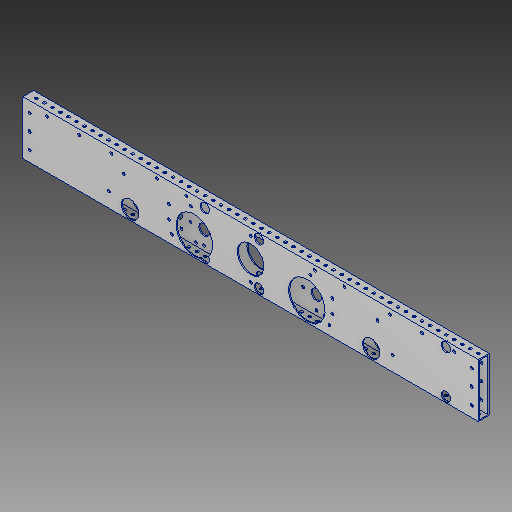
# Autodesk Inventor part: Side Extrusion
Saved by Autodesk Inventor 2019.4 (Build 234330000, 330)
## iProperties
Created: 2019-11-02
Part Number: Side Extrusion
Material: Aluminum 6061
Document SubType Name: Modeling
Designer: admin
Density: 2.7 g/cm^3
Appearance: Aluminum - Flat
Mass: 944.762 g
Surface Area: 3612.85 cm^2
Volume: 349.912 cm^3
Author: admin
Autodesk Inventor part; units mm, degrees
ref_plane "YZ Plane" through (0, 0, 0) normal (1, 0, 0) x (0, 1, 0)
ref_plane "XZ Plane" through (0, 0, 0) normal (0, 1, 0) x (-1, 0, 0)
ref_plane "XY Plane" through (0, 0, 0) normal (0, 0, 1) x (1, 0, 0)
sketch "Sketch1" plane through (0, 0, 0) normal (1, 0, 0) x (0, 1, 0)
  line L0 (-50, 10) -> (50, 10)
  line L1 (50, 10) -> (50, -10)
  line L2 (50, -10) -> (-50, -10)
  line L3 (-50, -10) -> (-50, 10)
  line L4 (-50, 10) -> (50, -10) construction
  line L5 (50, 10) -> (-50, -10) construction
  line L6 (48, -8) -> (48, 8)
  line L7 (48, 8) -> (-48, 8)
  line L8 (-48, 8) -> (-48, -8)
  line L9 (-48, -8) -> (48, -8)
  point P0 (0, 0)
  dimension "d0" = 100
  dimension "d1" = 20
  dimension "d2" = 2
  constraints: 20 end point, 4 parallel, 2 midpoint, 2 perpendicular, 1 horizontal, 3 other
  measures "d0" distance of L1.end L2.end
  measures "d1" distance of L0.end L1.end
  measures "d2" distance between parallel lines of L1 L6
extrude "Extrusion1" add sketch "Sketch1" along normal blind 850
sketch "Sketch2" plane through (0, -50, 10) normal (0, 0, -1) x (-1, 0, 0)
  circle A0 centre (-200, 18.3) radius 16.3
  line L0 (0, 0) -> (-850, 0) projected
  line L1 (0, 100) -> (0, 0) projected
  line L2 (0, 100) -> (-850, 100) projected
  line L3 (0, 0) -> (-850, 0) projected
  circle A1 centre (-650, 18.3) radius 16.3
  line L4 (-850, 100) -> (-850, 0) projected
  point P0 (0, 50)
  dimension "d5" = 32.6
  dimension "d9" = 200
  dimension "d113" = 200
  constraints: 2 centre point
  measures "d5" diameter of A0
  measures "d9" distance from line of L1 A0.centre
  measures "d113" distance from line of L4 A1.centre
extrude "Extrusion2" cut sketch "Sketch2" along normal blind 2 contours A0 | A1
sketch "Sketch3" plane through (0, -50, 10) normal (0, 0, 1) x (1, 0, 0)
  circle A0 centre (320, 36) radius 34
  line L0 (0, 0) -> (0, 100) projected
  line L1 (0, 0) -> (850, 0) projected
  line L2 (425, 100) -> (425, 0)
  circle A1 centre (530, 36) radius 34
  point P0 (0, 50)
  dimension "d10" = 68
  dimension "d11" = 320
  dimension "d12" = 36
  constraints: 2 centre point, 2 end point, 1 midpoint, 1 symmetric about line, 1 other
  measures "d10" diameter of A0
  measures "d11" distance from line of L0 A0.centre
  measures "d12" distance from line of A0.centre L1
extrude "Extrusion3" cut sketch "Sketch3" against normal blind 2
sketch "Sketch4" plane through (0, -50, -10) normal (0, 0, -1) x (-1, 0, 0)
  circle A0 centre (-200, 18.3) radius 16.3 construction
  circle A1 centre (-200, 18.3) radius 16.3 construction
  circle A2 centre (-200, 18.3) radius 12.3
  line L0 (0, 0) -> (-850, 0) projected
  line L1 (-425, 0) -> (-425, 100)
  line L2 (0, 100) -> (-850, 100) projected
  circle A3 centre (-650, 18.3) radius 12.3
  point P0 (0, 50)
  point P1 (-200, 2)
  dimension "d17" = 24.6
  constraints: 2 centre point, 2 end point, 2 midpoint, 1 coincident, 1 symmetric about line, 1 vertical alignment, 1 other
  measures "d17" diameter of A2
extrude "Extrusion4" cut sketch "Sketch4" against normal blind 2
sketch "Sketch5" plane through (0, -50, -10) normal (0, 0, -1) x (-1, 0, 0)
  circle A0 centre (-216, 18.3) radius 2.25
  circle A1 centre (-200, 18.3) radius 12.3 projected
  line L0 (-200, 18.3) -> (-216, 18.3) construction
  circle A2 centre (-200, 34.3) radius 2.25
  circle A3 centre (-184, 18.3) radius 2.25
  line L1 (0, 100) -> (-850, 100) projected
  line L2 (-425, 100) -> (-425, 0)
  line L3 (0, 0) -> (-850, 0) projected
  circle A4 centre (-634, 18.3) radius 2.25
  circle A5 centre (-650, 34.3) radius 2.25
  circle A6 centre (-666, 18.3) radius 2.25
  point P0 (0, 50)
  dimension "d18" = 4.5
  dimension "d21" = 16
  dimension "d24" = 180
  constraints: 6 centre point, 4 end point, 3 symmetric about line, 2 midpoint, 1 horizontal, 8 other
  measures "d18" diameter of A0
  measures "d21" distance of L0.start L0.end
extrude "Extrusion5" cut sketch "Sketch5" against normal blind 2 contours A0 | A2 | A3 | A4 | A5 | A6
sketch "Sketch6" plane through (0, -50, -10) normal (0, 0, -1) x (-1, 0, 0)
  circle A0 centre (-320, 36) radius 10
  line L0 (0, 0) -> (-850, 0)
  line L1 (0, 100) -> (0, 0)
  circle A1 centre (-320, 36) radius 25.4
  circle A2 centre (-320, 61.4) radius 2.75
  circle A3 centre (-345.4, 36) radius 2.75
  circle A4 centre (-320, 10.6) radius 2.75
  circle A5 centre (-294.6, 36) radius 2.75
  line L2 (-253.104106, 23.400764) -> (-232.795044, 42.581828)
  arc A6 (-232.795044, 42.581828) -> (-221.861202, 43.200848) centre (-228.087042, 56.296226) ccw
  line L3 (-221.861202, 43.200848) -> (-214.225519, 31.637858)
  arc A7 (-214.225519, 31.637858) -> (-219.215212, 21.622298) centre (-200.000275, 18.300226) ccw
  line L4 (-219.215212, 21.622298) -> (-250.723733, 18.236908)
  arc A8 (-253.104106, 23.400764) -> (-250.723733, 18.236908) centre (-251.04422, 21.21974) ccw
  line L5 (-211.588609, 53.460841) -> (-194.873767, 53.460841)
  arc A9 (-192.370348, 52.113987) -> (-194.873767, 53.460841) centre (-194.873767, 50.460841) ccw
  line L6 (-192.370348, 52.113987) -> (-179.138449, 32.076445)
  arc A10 (-175.035626, 16.971193) -> (-179.138449, 32.076445) centre (-200.000275, 18.300226) ccw
  arc A11 (-178.031384, 14.130677) -> (-175.035626, 16.971193) centre (-178.031384, 17.130677) ccw
  arc A12 (-180.528551, 17.250469) -> (-178.031384, 14.130677) centre (-177.532902, 17.088968) ccw
  arc A13 (-180.528551, 17.250469) -> (-207.029984, 36.489046) centre (-200.000275, 18.300226) ccw
  arc A14 (-210.536046, 37.520558) -> (-207.029984, 36.489046) centre (-208.111478, 39.287326) ccw
  line L7 (-210.536046, 37.520558) -> (-215.905928, 44.889746)
  arc A15 (-215.985191, 48.309036) -> (-215.905928, 44.889746) centre (-213.481359, 46.656514) ccw
  arc A16 (-215.985191, 48.309036) -> (-214.416912, 51.461193) centre (-228.087042, 56.296226) ccw
  arc A17 (-211.588609, 53.460841) -> (-214.416912, 51.461193) centre (-211.588609, 50.460841) ccw
  line L8 (-284.480973, 40.652695) -> (-284.222617, 32.873773)
  arc A18 (-288.433061, 30.029957) -> (-284.222617, 32.873773) centre (-287.220964, 32.774191) ccw
  line L9 (-288.433061, 30.029957) -> (-290.947932, 31.140747)
  arc A19 (-305.816396, 47.278292) -> (-290.947932, 31.140747) centre (-279.837042, 56.296226) ccw
  arc A20 (-302.982285, 51.262067) -> (-305.816396, 47.278292) centre (-302.982285, 48.262067) ccw
  line L10 (-302.982285, 51.262067) -> (-295.383819, 51.262067)
  arc A21 (-292.718657, 49.639351) -> (-295.383819, 51.262067) centre (-295.383819, 48.262067) ccw
  arc A22 (-292.718657, 49.639351) -> (-286.169215, 43.251933) centre (-279.837042, 56.296226) ccw
  arc A23 (-284.480973, 40.652695) -> (-286.169215, 43.251933) centre (-287.479319, 40.553113) ccw
  arc A24 (-214.415926, -2.662574) -> (-211.443355, 2.510802) centre (-213.203829, 0.08166) ccw
  line L11 (-214.415926, -2.662574) -> (-233.317299, 5.685948)
  arc A25 (-232.531596, 11.399725) -> (-233.317299, 5.685948) centre (-232.105201, 8.430182) ccw
  line L12 (-232.531596, 11.399725) -> (-221.353674, 13.004754)
  arc A26 (-218.137012, 11.137213) -> (-221.353674, 13.004754) centre (-220.927279, 10.035211) ccw
  arc A27 (-218.137012, 11.137213) -> (-211.443355, 2.510802) centre (-200.000275, 18.300226) ccw
  arc A28 (-192.284251, 0.391765) -> (-193.492561, -1.479829) centre (-191.492864, -1.445001) ccw
  arc A29 (-192.284251, 0.391765) -> (-186.463613, 4.264244) centre (-200.000275, 18.300226) ccw
  arc A30 (-185.075238, 4.824656) -> (-186.463613, 4.264244) centre (-185.075238, 2.824656) ccw
  arc A31 (-181.505821, 1.478954) -> (-182.985377, 4.824656) centre (-182.985377, 2.824656) ccw
  arc A32 (-190.722566, -4.914513) -> (-181.505821, 1.478954) centre (-200.000275, 18.300226) ccw
  line L13 (-284.545044, 79.552122) -> (-284.545044, 72.007264)
  arc A33 (-286.223672, 69.313943) -> (-284.545044, 72.007264) centre (-287.545044, 72.007264) ccw
  arc A34 (-286.223672, 69.313943) -> (-292.718657, 62.9531) centre (-279.837042, 56.296226) ccw
  arc A35 (-295.383819, 61.330385) -> (-292.718657, 62.9531) centre (-295.383819, 64.330385) ccw
  line L14 (-295.383819, 61.330385) -> (-302.982285, 61.330385)
  arc A36 (-305.816396, 65.314159) -> (-302.982285, 61.330385) centre (-302.982285, 64.330385) ccw
  arc A37 (-288.48888, 82.399783) -> (-305.816396, 65.314159) centre (-279.837042, 56.296226) ccw
  arc A38 (-284.545044, 79.552122) -> (-288.48888, 82.399783) centre (-287.545044, 79.552122) ccw
  line L15 (-228.585112, 83.796226) -> (-228.087042, 83.796226)
  arc A39 (-205.139033, 71.450067) -> (-228.087042, 83.796226) centre (-228.087042, 56.296226) ccw
  line L16 (-205.139033, 71.450067) -> (-200.077204, 63.784757)
  arc A40 (-202.580623, 59.131611) -> (-200.077204, 63.784757) centre (-202.580623, 62.131611) ccw
  line L17 (-202.580623, 59.131611) -> (-211.588609, 59.131611)
  arc A41 (-214.416912, 61.131259) -> (-211.588609, 59.131611) centre (-211.588609, 62.131611) ccw
  arc A42 (-214.416912, 61.131259) -> (-226.31563, 70.687616) centre (-228.087042, 56.296226) ccw
  arc A43 (-228.763039, 72.624992) -> (-226.31563, 70.687616) centre (-225.949131, 73.665144) ccw
  line L18 (-228.763039, 72.624992) -> (-231.399021, 79.756073)
  arc A44 (-228.585112, 83.796226) -> (-231.399021, 79.756073) centre (-228.585112, 80.796226) ccw
  line L19 (-265.847311, 52.483428) -> (-242.076773, 52.483428)
  arc A45 (-242.076773, 52.483428) -> (-238.294776, 45.998062) centre (-228.087042, 56.296226) ccw
  line L20 (-238.294776, 45.998062) -> (-267.247335, 24.919745)
  arc A46 (-271.929703, 26.642844) -> (-267.247335, 24.919745) centre (-269.013051, 27.34508) ccw
  line L21 (-271.929703, 26.642844) -> (-275.109946, 39.851591)
  arc A47 (-273.50365, 43.252524) -> (-275.109946, 39.851591) centre (-272.193293, 40.553828) ccw
  arc A48 (-273.50365, 43.252524) -> (-265.847311, 52.483428) centre (-279.837042, 56.296226) ccw
  line L22 (-244.206464, 60.109024) -> (-263.717619, 60.109024)
  arc A49 (-266.480949, 61.941115) -> (-263.717619, 60.109024) centre (-263.717619, 63.109024) ccw
  arc A50 (-266.480949, 61.941115) -> (-271.460037, 68.131588) centre (-279.837042, 56.296226) ccw
  arc A51 (-272.726863, 70.580283) -> (-271.460037, 68.131588) centre (-269.726863, 70.580283) ccw
  line L23 (-272.726863, 70.580283) -> (-272.726863, 80.796226)
  arc A52 (-269.726863, 83.796226) -> (-272.726863, 80.796226) centre (-269.726863, 80.796226) ccw
  line L24 (-269.726863, 83.796226) -> (-241.992001, 83.796226)
  arc A53 (-239.348967, 82.215513) -> (-241.992001, 83.796226) centre (-241.992001, 80.796226) ccw
  line L25 (-239.348967, 82.215513) -> (-234.298397, 72.810208)
  arc A54 (-235.423535, 68.803259) -> (-234.298397, 72.810208) centre (-236.94143, 71.390921) ccw
  arc A55 (-235.423535, 68.803259) -> (-241.443135, 61.941115) centre (-228.087042, 56.296226) ccw
  arc A56 (-244.206464, 60.109024) -> (-241.443135, 61.941115) centre (-244.206464, 63.109024) ccw
  circle A57 centre (-188.087042, 69.219) radius 2.75
  circle A58 centre (-277.837042, 16.582759) radius 2.75
  circle A59 centre (-250.087042, 92.776017) radius 2.75
  circle A60 centre (-160.000305, 27.300362) radius 2.75
  circle A61 centre (-313.422276, 79.81286) radius 2.75
  circle A62 centre (-200.000275, 18.300226) radius 9.5
  circle A63 centre (-228.087042, 56.296226) radius 9.5
  circle A64 centre (-279.837042, 56.296226) radius 9.5
  arc A65 (-244.094047, 93.065872) -> (-256.080036, 92.486162) centre (-250.087042, 92.776017) ccw
  line L26 (-256.080036, 92.486162) -> (-281.527863, 91.255361)
  arc A66 (-281.527863, 91.255361) -> (-302.063851, 83.332663) centre (-279.837042, 56.296226) ccw
  line L27 (-312.063851, 85.657061) -> (-302.063851, 83.332663)
  arc A67 (-312.063851, 85.657061) -> (-318.449419, 76.537524) centre (-313.422276, 79.81286) ccw
  line L28 (-312.844999, 67.935588) -> (-318.449419, 76.537524)
  arc A68 (-312.844999, 67.935588) -> (-294.877776, 24.692804) centre (-279.837042, 56.296226) ccw
  line L29 (-294.877776, 24.692804) -> (-283.254771, 19.16117)
  arc A69 (-283.254771, 19.16117) -> (-272.419312, 14.004347) centre (-277.837042, 16.582759) ccw
  line L30 (-272.419312, 14.004347) -> (-215.041009, -13.303196)
  arc A70 (-215.041009, -13.303196) -> (-165.000275, 18.300352) centre (-200.000275, 18.300226) ccw
  line L31 (-160.000305, 21.300362) -> (-162.000275, 21.300362)
  arc A71 (-160.000305, 21.300362) -> (-156.580779, 22.370166) centre (-160.000305, 27.300362) ccw
  arc A72 (-169.897664, 36.156116) -> (-170.793719, 37.586933) centre (-200.000275, 18.300226) ccw
  line L32 (-170.793719, 37.586933) -> (-184.354376, 58.122326)
  arc A73 (-187.633238, 75.201814) -> (-191.393334, 74.225838) centre (-188.087042, 69.219) ccw
  line L33 (-195.5499, 75.076111) -> (-196.794303, 76.960555)
  arc A74 (-196.794303, 76.960555) -> (-229.898636, 93.752442) centre (-228.087042, 56.296226) ccw
  line L34 (-229.898636, 93.752442) -> (-244.094047, 93.065872)
  line L35 (0, 100) -> (-850, 100)
  line L36 (-425, 100) -> (-425, 0)
  circle A75 centre (-530, 61.4) radius 2.75
  circle A76 centre (-504.6, 36) radius 2.75
  circle A77 centre (-530, 10.6) radius 2.75
  circle A78 centre (-555.4, 36) radius 2.75
  circle A79 centre (-661.912958, 69.219) radius 2.75
  circle A80 centre (-572.162958, 16.582759) radius 2.75
  circle A81 centre (-599.912958, 92.776017) radius 2.75
  circle A82 centre (-689.999695, 27.300362) radius 2.75
  circle A83 centre (-536.577724, 79.81286) radius 2.75
  line L37 (-156.580779, 22.370166) -> (-137.281762, 35.755737)
  arc A84 (-137.281762, 35.755737) -> (-147.167505, 72.132439) centre (-148.680183, 52.189726) ccw
  line L38 (-147.167505, 72.132439) -> (-187.633238, 75.201814)
  arc A85 (-195.5499, 75.076111) -> (-191.393334, 74.225838) centre (-193.046481, 76.729257) ccw
  arc A86 (-162.000275, 21.300362) -> (-165.000275, 18.300352) centre (-162.000275, 18.300362) ccw
  circle A87 centre (-148.680183, 52.189726) radius 10.5
  circle A88 centre (-163.234444, 48.560195) radius 1.65
  arc A89 (-181.624055, 62.766879) -> (-184.354376, 58.122326) centre (-181.850957, 59.775472) ccw
  line L39 (-181.624055, 62.766879) -> (-170.444252, 61.918877)
  arc A90 (-167.802767, 58.048634) -> (-170.444252, 61.918877) centre (-170.671154, 58.92747) ccw
  arc A91 (-167.802767, 58.048634) -> (-164.446092, 39.883788) centre (-148.680183, 52.189726) ccw
  arc A92 (-165.101215, 35.572799) -> (-164.446092, 39.883788) centre (-166.810978, 38.037897) ccw
  line L40 (-165.101215, 35.572799) -> (-165.607677, 35.221523)
  arc A93 (-169.897664, 36.156116) -> (-165.607677, 35.221523) centre (-167.31744, 37.686621) ccw
  circle A94 centre (-144.546319, 66.608851) radius 1.65
  circle A95 centre (-138.259787, 41.400132) radius 1.65
  circle A96 centre (-530, 36) radius 10
  line L41 (-193.464479, -3.092162) -> (-193.492561, -1.479829)
  line L42 (-185.075238, 4.824656) -> (-182.985377, 4.824656)
  arc A97 (-193.464479, -3.092162) -> (-190.722566, -4.914513) centre (-191.464783, -3.057334) ccw
  point P0 (0, 50)
  point P1 (-200.000275, 18.300226)
  point P2 (-200.000275, 18.300226)
  point P3 (-200.000275, 18.300226)
  point P4 (-200.000275, 18.300226)
  point P5 (-162.000275, 18.300362)
  point P6 (-167.31744, 37.686621)
  point P7 (-200.000275, 18.300226)
  dimension "d31" = 50.8
  dimension "d28" = 20
  dimension "d29" = 36
  dimension "d30" = 320
  dimension "d32" = 5.5
  dimension "d35" = 360
  dimension "d46" = 36
  constraints: 15 centre point, 10 symmetric about line, 2 end point, 2 midpoint, 1 coincident, 1 vertical alignment, 21 other
  measures "d28" diameter of A0
  measures "d29" distance from line of L0 A0.centre
  measures "d30" distance from line of L1 A0.centre
  measures "d32" diameter of A2
  measures "d46" distance from line of L0 A3.centre
extrude "Extrusion6" cut sketch "Sketch6" against normal blind 50 contours A0 | A2 A1 | A1 A2 | A4 A1 | A1 A4 | A5 A1 | A1 A5 A19 | A5 A19 | A3 A1 | A1 A3 | A57 | A58 | A59 | A60 | A61 | A75 | A76 | A77 | A78 | A79 | A80 | A81 | A82 | A83 | A96 picked at (-296.100043, 35.292408)
sketch "Sketch7" plane through (0, -50, -10) normal (0, 0, -1) x (-1, 0, 0)
  circle A0 centre (-228.087, 56.296) radius 10.5
  line L0 (0, 100) -> (-850, 100) projected
  line L1 (0, 100) -> (0, 0) projected
  circle A1 centre (-279.787, 56.296) radius 10.5
  line L2 (-228.087, 56.296) -> (-279.787, 56.296) construction
  line L3 (-425, 100) -> (-425, 0)
  circle A2 centre (-621.913, 56.296) radius 10.5
  circle A3 centre (-570.213, 56.296) radius 10.5
  point P0 (0, 50)
  dimension "d39" = 43.704
  dimension "d40" = 228.087
  dimension "d41" = 21
  dimension "d44" = 21
  dimension "d45" = 51.7
  constraints: 4 centre point, 4 end point, 2 symmetric about line, 1 horizontal, 1 midpoint, 1 vertical, 2 other
  measures "d39" distance from line of L0 L2.start
  measures "d40" distance from line of L1 L2.start
  measures "d41" diameter of A0
  measures "d44" diameter of A1
  measures "d45" distance of L2.start L2.end
extrude "Extrusion7" cut sketch "Sketch7" against normal up to surface (2 mm away)
sketch "Sketch8" plane through (0, -50, -10) normal (0, 0, -1) x (-1, 0, 0)
  circle A0 centre (-425, 87.5) radius 2.75
  circle A1 centre (-545, 92) radius 2.75
  circle A2 centre (-685, 90.5) radius 2.75
  circle A3 centre (-805, 90.5) radius 2.75
  circle A4 centre (-745, 90.5) radius 2.75
  circle A5 centre (-837.5, 50) radius 2.75
  circle A6 centre (-837.5, 80) radius 2.75
  circle A7 centre (-837.5, 20) radius 2.75
  circle A8 centre (-425, 12.5) radius 2.75
  circle A9 centre (-545, 8) radius 2.75
  line L0 (-850, 0) -> (-850, 100) construction
  line L1 (0, 100) -> (-850, 100) construction
  line L2 (0, 0) -> (-850, 0) construction
  line L3 (0, 0) -> (-850, 0) construction
  line L4 (-425, 0) -> (-425, 100)
  circle A10 centre (-305, 92) radius 2.75
  circle A11 centre (-165, 90.5) radius 2.75
  circle A12 centre (-45, 90.5) radius 2.75
  circle A13 centre (-105, 90.5) radius 2.75
  circle A14 centre (-12.5, 50) radius 2.75
  circle A15 centre (-12.5, 80) radius 2.75
  circle A16 centre (-12.5, 20) radius 2.75
  circle A17 centre (-305, 8) radius 2.75
  line L5 (0, 0) -> (0, 100) construction
  line L6 (0, 0) -> (-850, 0) construction
  line L7 (0, 0) -> (-850, 0) projected
  line L8 (0, 100) -> (0, 0) projected
  line L9 (-850, 0) -> (-850, 100) projected
  dimension "d49" = 5.5
  dimension "d50" = 5.5
  dimension "d51" = 5.5
  dimension "d52" = 12.5
  dimension "d53" = 12.5
  dimension "d54" = 12.5
  dimension "d55" = 20
  dimension "d56" = 20
  dimension "d57" = 50
  dimension "d58" = 45
  dimension "d59" = 105
  dimension "d60" = 60
  dimension "d61" = 9.5
  dimension "d62" = 9.5
  dimension "d63" = 9.5
  dimension "d64" = 5.5
  dimension "d65" = 5.5
  dimension "d66" = 5.5
  dimension "d80" = 12.5
  dimension "d81" = 8
  dimension "d84" = 8
  dimension "d88" = 305
  dimension "d89" = 305
  dimension "d90" = 12.5
  dimension "d91" = 100
  dimension "d133" = 90
  constraints: 18 centre point, 14 end point, 8 symmetric about line, 4 equal radius, 3 collinear, 3 point on line, 2 midpoint, 8 other
  measures "d49" diameter of A6
  measures "d50" diameter of A5
  measures "d51" diameter of A7
  measures "d52" distance from line of L0 A7.centre
  measures "d53" distance from line of L0 A5.centre
  measures "d54" distance from line of L0 A6.centre
  measures "d55" distance from line of L1 A6.centre
  measures "d56" distance from line of L2 A7.centre
  measures "d57" distance from line of L1 A5.centre
  measures "d58" distance from line of L0 A3.centre
  measures "d59" distance from line of L0 A4.centre
  measures "d60" distance of A4.centre A2.centre
  measures "d61" distance from line of L1 A3.centre
  measures "d62" distance from line of L1 A4.centre
  measures "d63" distance from line of L1 A2.centre
  measures "d64" diameter of A3
  measures "d65" diameter of A4
  measures "d66" diameter of A2
  measures "d80" distance from line of L2 A8.centre
  measures "d81" distance from line of L2 A9.centre
  measures "d84" distance from line of L1 A1.centre
  measures "d88" distance from line of L0 A1.centre
  measures "d89" distance from line of L0 A9.centre
  measures "d90" distance from line of L1 A0.centre
  measures "d91" distance between parallel lines of L1 L3
  measures "d133" angle of L1 L5
extrude "Extrusion8" cut sketch "Sketch8" against normal blind 50
sketch "Sketch9" plane through (0, -50, 10) normal (0, 0, 1) x (1, 0, 0)
  circle A0 centre (272.5, 62.5) radius 2.75
  circle A1 centre (272.5, 37.5) radius 2.75
  line L0 (0, 100) -> (850, 100) projected
  line L1 (425, 100) -> (425, 0)
  line L2 (0, 0) -> (850, 0) projected
  line L3 (0, 0) -> (0, 100) projected
  circle A2 centre (577.5, 62.5) radius 2.75
  circle A3 centre (577.5, 37.5) radius 2.75
  point P0 (0, 50)
  dimension "d94" = 5.5
  dimension "d95" = 5.5
  dimension "d96" = 272.5
  dimension "d97" = 272.5
  dimension "d98" = 37.5
  dimension "d99" = 37.5
  constraints: 4 centre point, 2 end point, 2 midpoint, 2 symmetric about line, 2 other
  measures "d94" diameter of A0
  measures "d95" diameter of A1
  measures "d96" distance from line of L3 A0.centre
  measures "d97" distance from line of L3 A1.centre
  measures "d98" distance from line of L2 A1.centre
  measures "d99" distance from line of L0 A0.centre
extrude "Extrusion9" cut sketch "Sketch9" against normal blind 5 contours A0 | A1 | A2 | A3
sketch "Sketch10" plane through (0, 50, 10) normal (0, 1, 0) x (1, 0, 0)
  line L0 (0, 20) -> (850, 20) projected
  circle A0 centre (15, 10) radius 2.75
  line L1 (15, 10) -> (0, 10) construction
  circle A1 centre (30, 10) radius 2.75
  circle A2 centre (45, 10) radius 2.75
  circle A3 centre (60, 10) radius 2.75
  circle A4 centre (75, 10) radius 2.75
  circle A5 centre (90, 10) radius 2.75
  circle A6 centre (105, 10) radius 2.75
  circle A7 centre (120, 10) radius 2.75
  circle A8 centre (135, 10) radius 2.75
  circle A9 centre (150, 10) radius 2.75
  circle A10 centre (165, 10) radius 2.75
  circle A11 centre (180, 10) radius 2.75
  circle A12 centre (195, 10) radius 2.75
  circle A13 centre (210, 10) radius 2.75
  circle A14 centre (225, 10) radius 2.75
  circle A15 centre (240, 10) radius 2.75
  circle A16 centre (255, 10) radius 2.75
  circle A17 centre (270, 10) radius 2.75
  circle A18 centre (285, 10) radius 2.75
  circle A19 centre (300, 10) radius 2.75
  circle A20 centre (315, 10) radius 2.75
  circle A21 centre (330, 10) radius 2.75
  circle A22 centre (345, 10) radius 2.75
  circle A23 centre (360, 10) radius 2.75
  circle A24 centre (375, 10) radius 2.75
  circle A25 centre (390, 10) radius 2.75
  circle A26 centre (405, 10) radius 2.75
  circle A27 centre (420, 10) radius 2.75
  circle A28 centre (435, 10) radius 2.75
  circle A29 centre (450, 10) radius 2.75
  circle A30 centre (465, 10) radius 2.75
  circle A31 centre (480, 10) radius 2.75
  circle A32 centre (495, 10) radius 2.75
  circle A33 centre (510, 10) radius 2.75
  circle A34 centre (525, 10) radius 2.75
  circle A35 centre (540, 10) radius 2.75
  circle A36 centre (555, 10) radius 2.75
  circle A37 centre (570, 10) radius 2.75
  circle A38 centre (585, 10) radius 2.75
  circle A39 centre (600, 10) radius 2.75
  circle A40 centre (615, 10) radius 2.75
  circle A41 centre (630, 10) radius 2.75
  circle A42 centre (645, 10) radius 2.75
  circle A43 centre (660, 10) radius 2.75
  circle A44 centre (675, 10) radius 2.75
  circle A45 centre (690, 10) radius 2.75
  circle A46 centre (705, 10) radius 2.75
  circle A47 centre (720, 10) radius 2.75
  circle A48 centre (735, 10) radius 2.75
  circle A49 centre (750, 10) radius 2.75
  circle A50 centre (765, 10) radius 2.75
  circle A51 centre (780, 10) radius 2.75
  circle A52 centre (795, 10) radius 2.75
  circle A53 centre (810, 10) radius 2.75
  circle A54 centre (825, 10) radius 2.75
  circle A55 centre (840, 10) radius 2.75
  dimension "d102" = 5.5
  dimension "d103" = 15
  dimension "d106" = 15
  constraints: 56 centre point, 2 end point, 2 horizontal, 110 other
  measures "d102" diameter of A0
  measures "d103" distance of L1.start L1.end
  measures "d106" distance of L1.start A1.centre
extrude "Extrusion10" cut sketch "Sketch10" against normal through all
sketch "Sketch11" plane through (0, -50, -10) normal (0, 0, -1) x (-1, 0, 0)
  point P0 (0, 50)
sketch "Sketch12" plane through (0, -50, -10) normal (0, 0, -1) x (-1, 0, 0)
  circle A0 centre (-577.5, 62.5) radius 2.75 projected
  circle A1 centre (-577.5, 62.5) radius 2.75 projected
  circle A2 centre (-577.5, 37.5) radius 2.75 projected
  circle A3 centre (-577.5, 37.5) radius 2.75 projected
  circle A4 centre (-272.5, 62.5) radius 2.75 projected
  circle A5 centre (-272.5, 62.5) radius 2.75 projected
  circle A6 centre (-272.5, 37.5) radius 2.75 projected
  circle A7 centre (-272.5, 37.5) radius 2.75 projected
  circle A8 centre (-577.5, 37.5) radius 7.5
  circle A9 centre (-272.5, 37.5) radius 7.5
  point P0 (0, 50)
  dimension "d114" = 15
  dimension "d115" = 15
  constraints: 2 centre point, 2 coincident
  measures "d114" diameter of A8
  measures "d115" diameter of A9
extrude "Extrusion11" cut sketch "Sketch12" against normal blind 2 contours A2 | A6 | A8 | A9
sketch "Sketch13" plane through (0, -50, -10) normal (0, 0, -1) x (-1, 0, 0)
  circle A0 centre (-789.4, 90) radius 2.75 projected
  circle A1 centre (-789.5, 10) radius 2.75 projected
  circle A2 centre (-440.6, 90) radius 2.75 projected
  circle A3 centre (-440.6, 10) radius 2.75 projected
  circle A4 centre (-339.4, 90) radius 2.75 projected
  circle A5 centre (-339.4, 10) radius 2.75 projected
  point P0 (0, 50)
extrude "Extrusion12" cut sketch "Sketch13" against normal through all
sketch "Sketch14" plane through (0, -50, 10) normal (0, 0, 1) x (1, 0, 0)
  circle A0 centre (339.4, 90) radius 2.75
  circle A1 centre (789.4, 90) radius 2.75
  circle A2 centre (789.5, 10) radius 2.75
  circle A3 centre (440.6, 10) radius 2.75
  circle A4 centre (440.6, 90) radius 2.75
  circle A5 centre (339.4, 90) radius 2.75
  circle A6 centre (339.4, 10) radius 2.75
  circle A7 centre (339.4, 90) radius 8.75
  circle A8 centre (339.4, 10) radius 8.75
  circle A9 centre (440.6, 10) radius 8.75
  circle A10 centre (440.6, 90) radius 8.75
  circle A11 centre (789.4, 90) radius 8.75
  circle A12 centre (789.5, 10) radius 8.75
  point P0 (0, 50)
extrude "Extrusion13" cut sketch "Sketch14" against normal blind 3
sketch "Sketch15" plane through (0, -50, -10) normal (0, 0, -1) x (-1, 0, 0)
  circle A0 centre (-425, 50) radius 25
  line L0 (0, 0) -> (-850, 0) projected
  line L1 (0, 100) -> (0, 0) projected
  point P0 (0, 50)
  dimension "d128" = 50
  dimension "d129" = 50
  dimension "d130" = 425
  constraints: 1 centre point
  measures "d128" diameter of A0
  measures "d129" distance from line of L0 A0.centre
  measures "d130" distance from line of L1 A0.centre
extrude "Extrusion14" cut sketch "Sketch15" against normal blind 65.5
sketch "Sketch16" plane through (0, -50, -10) normal (0, 0, -1) x (-1, 0, 0)
  circle A0 centre (-425, 12.5) radius 2.75 projected
  circle A1 centre (-425, 12.5) radius 7.75
  point P0 (0, 50)
  dimension "d134" = 5
  constraints: 1 centre point
  measures "d134" radial gap between concentric circles of A0 A1
extrude "Extrusion15" cut sketch "Sketch16" against normal blind 2
sketch "Sketch17" plane through (0, -50, -10) normal (0, 0, -1) x (-1, 0, 0)
  circle A0 centre (-805, 90.5) radius 2.75 projected
  circle A1 centre (-805, 90.5) radius 6.75
  point P0 (0, 50)
  dimension "d137" = 4
  constraints: 1 centre point
  measures "d137" radial gap between concentric circles of A0 A1
extrude "Extrusion16" cut sketch "Sketch17" against normal blind 2
equation "\"d97\" = d96"
equation "\"d98\" = d99"
body "Solid1"
